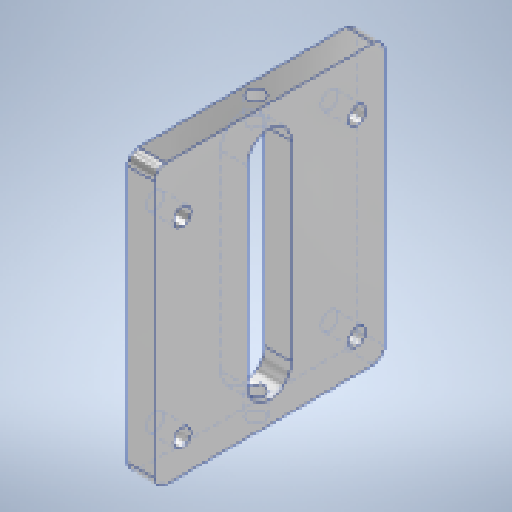
# Autodesk Inventor part: 2mm_double_for_pulley
Saved by Autodesk Inventor 2025 (Build 290162000, 162)
## iProperties
Created: 2025-02-24
Part Number: 2mm_double_for_pulley
Material: アルミニウム 6061
Document SubType Name: Modeling
Designer: Zhopa
Density: 2.7 g/cm^3
Appearance: アルミニウム - フラット
Mass: 23.8224 g
Surface Area: 51.9141 cm^2
Volume: 8.82309 cm^3
Author: Zhopa
Autodesk Inventor part; units mm, degrees
ref_plane "YZ Plane" through (0, 0, 0) normal (1, 0, 0) x (0, 1, 0)
ref_plane "XZ Plane" through (0, 0, 0) normal (0, 1, 0) x (-1, 0, 0)
ref_plane "XY Plane" through (0, 0, 0) normal (0, 0, 1) x (1, 0, 0)
sketch "Sketch1" plane through (0, 0, 0) normal (1, 0, 0) x (0, 1, 0)
  line L0 (-25.5, 21) -> (25.5, 21)
  line L1 (25.5, 21) -> (25.5, -21)
  line L2 (25.5, -21) -> (-25.5, -21)
  line L3 (-25.5, -21) -> (-25.5, 21)
  line L4 (-25.5, 21) -> (25.5, -21) construction
  line L5 (25.5, 21) -> (-25.5, -21) construction
  circle A0 centre (15.5, 16) radius 1.6
  circle A1 centre (15.5, -16) radius 1.6
  circle A2 centre (-19.5, -16) radius 1.6
  circle A3 centre (-19.5, 16) radius 1.6
  line L6 (17.5, 0) -> (-17.5, 0) construction
  line L7 (17.5, 4) -> (-17.5, 4)
  line L8 (-17.5, -4) -> (17.5, -4)
  arc A4 (17.5, -4) -> (17.5, 4) centre (17.5, 0) ccw
  arc A5 (-17.5, 4) -> (-17.5, -4) centre (-17.5, 0) ccw
  point P0 (0, 0)
  point P1 (-9.5, -16)
  point P2 (0, 0)
  point P3 (15.5, -48)
  point P4 (-19.5, -35.5845)
  dimension "d0" = 42
  dimension "d1" = 51
  dimension "d2" = 5
  dimension "d3" = 10
  dimension "d5" = 35
  dimension "d6" = 5
  dimension "d7" = 3.2
  dimension "d8" = 3.2
  dimension "d9" = 3.2
  dimension "d10" = 3.2
  dimension "d15" = 0
  dimension "d16" = 0
  dimension "d17" = 32
  dimension "d18" = 0
  dimension "d19" = 0
  dimension "d20" = 8
  dimension "d21" = 8
  dimension "d22" = 8
  dimension "d31" = 32
  constraints: 20 end point, 6 centre point, 4 point on circle, 4 tangent, 3 midpoint, 3 parallel, 2 horizontal, 1 coincident, 1 perpendicular
  measures "d0" distance of L0.end L1.end
  measures "d1" distance of L1.end L2.end
  measures "d2" distance from line of L0 point (15.5, 16)
  measures "d3" distance from line of point (15.5, 16) L1
  measures "d5" distance of point (15.5, 16) point (-19.5, 16)
  measures "d6" distance from line of L2 point (15.5, -16)
  measures "d7" diameter of A0
  measures "d8" diameter of A1
  measures "d9" diameter of A2
  measures "d10" diameter of A3
  measures "d15" distance of point (15.5, -16) A1.centre
  measures "d16" distance of point (-19.5, 16) A3.centre
  measures "d17" distance of point (-19.5, 16) A2.centre
  measures "d18" horizontal distance of A3.centre A2.centre
  measures "d19" horizontal distance of point (15.5, 16) A1.centre
  measures "d20" distance from line of L3 L6.end
  measures "d21" distance from line of L1 L6.start
  measures "d22" diameter of A5
  measures "d31" distance of point (15.5, -48) A1.centre
extrude "Extrusion1" add sketch "Sketch1" along normal blind 5
fillet "Fillet1" radius 2 4 edges at (2.5, 25.5, 21) (2.5, -25.5, 21) (2.5, -25.5, -21) (2.5, 25.5, -21)
sketch "Sketch2" plane through (0, 25.5, 19) normal (0, 1, 0) x (1, 0, 0)
  line L0 (0, 38) -> (0, 0) projected
  point P0 (0, 19)
  point P1 (2.5, 19)
  dimension "d23" = 2.5
  measures "d23" distance from line of point (2.5, 19) L0
hole "Hole1" at (2.5, 25.5, 0) direction (0, -1, 0) diameter 3 depth 80.45
body "Solid1"
